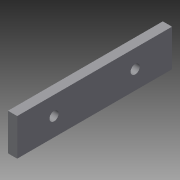
# Autodesk Inventor part: CURM_Caterpillar_wall
Saved by Autodesk Inventor 2015 (Build 190159000, 159)
## iProperties
Created: 2015-02-11
Part Number: CURM_Caterpillar_wall
Material: Generic
Document SubType Name: Modeling
Designer: Judson
Density: 1 g/cm^3
Appearance: Default
Author: Judson
Autodesk Inventor part; units mm, degrees
ref_plane "YZ Plane" through (0, 0, 0) normal (1, 0, 0) x (0, 1, 0)
ref_plane "XZ Plane" through (0, 0, 0) normal (0, 1, 0) x (-1, 0, 0)
ref_plane "XY Plane" through (0, 0, 0) normal (0, 0, 1) x (1, 0, 0)
sketch "Sketch1" plane through (0, 0, 0) normal (0, 1, 0) x (-1, 0, 0)
  line L0 (-3.9445, -24.4098) -> (-7.1195, -24.4098)
  line L1 (-7.1195, -24.4098) -> (-7.1195, 28.9302)
  line L2 (-7.1195, 28.9302) -> (-3.9445, 28.9302)
  line L3 (-3.9445, 28.9302) -> (-3.9445, -24.4098)
  point P0 (0, 0)
  dimension "d0" = 53.34
  dimension "d1" = 3.175
  constraints: 8 end point, 2 parallel, 1 horizontal, 1 perpendicular
  measures "d0" distance of L0.end L1.end
  measures "d1" distance of L1.end L2.end
extrude "Extrusion1" add sketch "Sketch1" along normal blind 12.7
sketch "Sketch2" plane through (7.1195, 0, 28.9302) normal (1, 0, 0) x (0, 0, -1)
  line L0 (0, 0) -> (53.34, 0) projected
  line L1 (53.34, 6.35) -> (40.64, 6.35)
  line L2 (40.64, 6.35) -> (40.64, 0)
  line L3 (40.64, 0) -> (53.34, 0)
  line L4 (53.34, 0) -> (53.34, 6.35)
  line L5 (53.34, 0) -> (53.34, 12.7) projected
  circle A0 centre (40.64, 6.35) radius 1.5875
  line L6 (53.34, 12.7) -> (0, 12.7) projected
  line L7 (26.67, 12.7) -> (26.67, 0)
  circle A1 centre (12.7, 6.35) radius 1.5875
  line L8 (0, 0) -> (0, 12.7) projected
  point P0 (28.9302, 0)
  dimension "d6" = 12.7
  dimension "d7" = 6.35
  dimension "d8" = 3.175
  dimension "d9" = 26.67
  dimension "d12" = 12.7
  dimension "d13" = 27.94
  constraints: 10 end point, 2 centre point, 2 midpoint, 2 parallel, 2 perpendicular, 1 coincident, 1 horizontal, 1 point on line, 1 symmetric about line, 1 other
  measures "d6" distance of L0.end L2.end
  measures "d7" distance of L0.end L1.start
  measures "d8" diameter of A0
  measures "d9" distance between parallel lines of L7 L5
  measures "d12" distance from line of L8 A1.centre
  measures "d13" distance of L1.end A1.centre
extrude "Extrusion2" cut sketch "Sketch2" against normal blind 3.175 contours A0 L1 L2 | L2 L1 A0 | A1
body "Solid1"
